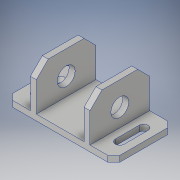
# Autodesk Inventor part: Block3
Saved by Autodesk Inventor 2019 (Build 230136000, 136)
## iProperties
Created: 2018-11-06
Part Number: Block3
Material: Aluminum 6061
Document SubType Name: Modeling
Designer: 2003189
Density: 2.7 g/cm^3
Appearance: Aluminum - Flat
Mass: 1550.39 g
Surface Area: 1099.84 cm^2
Volume: 574.22 cm^3
Author: 2003189
Autodesk Inventor part; units mm, degrees
ref_plane "YZ Plane" through (0, 0, 0) normal (1, 0, 0) x (0, 1, 0)
ref_plane "XZ Plane" through (0, 0, 0) normal (0, 1, 0) x (-1, 0, 0)
sketch "Sketch1" plane through (0, 0, 0) normal (0, 1, 0) x (-1, 0, 0)
  line L0 (0, 0) -> (-228.6, 0)
  line L1 (-228.6, 0) -> (-228.6, -127)
  line L2 (-228.6, -127) -> (0, -127)
  line L3 (0, -127) -> (0, 0)
  dimension "d0" = 228.6
  dimension "d1" = 127
  constraints: 8 end point, 2 parallel, 1 horizontal, 1 perpendicular
  measures "d0" distance of L2.end L1.end
  measures "d1" distance of L1.end L0.end
extrude "Extrusion1" add sketch "Sketch1" along normal blind 12.7
chamfer "Chamfer1" distance 12.7 angle 45 4 edges at (0, 6.35, 0) (228.6, 6.35, 0) (228.6, 6.35, -127) (0, 6.35, -127)
sketch "Sketch2" plane through (0, 12.7, 0) normal (0, 1, 0) x (1, 0, 0)
  line L0 (12.7, 0) -> (215.9, 0) projected
  line L1 (114.3, 0) -> (63.5, 0)
  line L2 (63.5, 0) -> (63.5, 127)
  line L3 (63.5, 127) -> (114.3, 127)
  line L4 (114.3, 127) -> (114.3, 0)
  line L5 (215.9, 127) -> (12.7, 127) projected
  line L6 (63.5, 0) -> (50.8, 0)
  line L7 (50.8, 0) -> (50.8, 127)
  line L8 (50.8, 127) -> (63.5, 127)
  line L9 (63.5, 127) -> (63.5, 0)
  line L10 (114.3, 0) -> (165.1, 0)
  line L11 (165.1, 0) -> (165.1, 127)
  line L12 (165.1, 127) -> (114.3, 127)
  line L13 (114.3, 127) -> (114.3, 0)
  line L14 (165.1, 0) -> (177.8, 0)
  line L15 (177.8, 0) -> (177.8, 127)
  line L16 (177.8, 127) -> (165.1, 127)
  line L17 (165.1, 127) -> (165.1, 0)
  point P0 (0, 0)
  dimension "d7" = 50.8
  dimension "d8" = 127
  dimension "d9" = 12.7
  dimension "d10" = 50.8
  dimension "d11" = 12.7
  constraints: 32 end point, 8 parallel, 4 horizontal, 4 perpendicular, 3 point on line, 1 midpoint
  measures "d7" distance of L2.end L3.end
  measures "d8" distance of L1.end L2.end
  measures "d9" distance of L7.end L8.end
  measures "d10" distance of L12.end L11.end
  measures "d11" distance of L16.end L15.end
extrude "Extrusion2" add sketch "Sketch2" along normal blind 88.9 contours L7 L5 L2 L0 | L11 L5 L15 L0
chamfer "Chamfer2" distance 25.4 angle 45 4 edges at (57.15, 101.6, 0) (57.15, 101.6, -127) (171.45, 101.6, 0) (171.45, 101.6, -127)
sketch "Sketch3" plane through (177.8, 12.7, 0) normal (1, 0, 0) x (0, 0, -1)
  line L0 (0, 0) -> (0, 63.5) projected
  line L1 (127, 0) -> (127, 63.5) projected
  line L2 (101.6, 88.9) -> (25.4, 88.9) projected
  line L3 (63.5, 88.9) -> (63.5, 38.1)
  circle A0 centre (63.5, 38.1) radius 19.05
  point P0 (0, -12.7)
  dimension "d17" = 50.8
  dimension "d18" = 38.1
  constraints: 2 end point, 1 centre point, 1 coincident, 1 midpoint, 1 vertical
  measures "d17" distance of L3.start L3.end
  measures "d18" diameter of A0
extrude "Extrusion3" cut sketch "Sketch3" against normal through all
sketch "Sketch6" plane through (0, 12.7, 0) normal (0, 1, 0) x (1, 0, 0)
  arc A0 (207.9625, 88.9) -> (198.4375, 88.9) centre (203.2, 88.9) ccw projected
  circle A1 centre (203.2, 88.9) radius 9.525
  arc A2 (198.4375, 38.1) -> (207.9625, 38.1) centre (203.2, 38.1) ccw projected
  circle A3 centre (203.2, 38.1) radius 9.525
  line L0 (193.675, 38.1) -> (193.675, 88.9)
  line L1 (212.725, 38.1) -> (212.725, 88.9)
  point P0 (0, 0)
  dimension "d31" = 19.05
  dimension "d32" = 19.05
  constraints: 4 end point, 4 point on circle, 2 centre point, 2 coincident, 1 parallel, 1 tangent, 1 vertical
  measures "d31" diameter of A1
  measures "d32" diameter of A3
extrude "Extrusion5" cut sketch "Sketch6" against normal blind 25.4
ref_plane "Work Plane1" through (114.3, 0, -114.3) normal (-1, 0, 0) x (0, 0, 1)
mirror "Mirror1" about plane through (114.3, 0, -114.3) normal (-1, 0, 0) of "Extrusion5"
body "Solid1"
